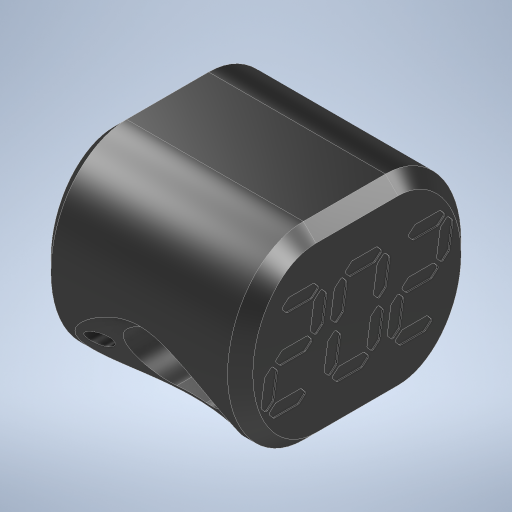
# Autodesk Inventor part: HeadCover
Saved by Autodesk Inventor 2024.2 (Build 282272000, 272)
## iProperties
Created: 2024-02-01
Part Number: HeadCover
Material: ABS Plastic
Document SubType Name: Modeling
Designer: Masato Kubotera
Density: 1.06 g/cm^3
Appearance: Glossy - Black
Mass: 122.703 g
Surface Area: 426.62 cm^2
Volume: 115.757 cm^3
Catalog Web Link: https://www.poly-maker.jp/polyterra-pla.html
Author: Masato Kubotera
Autodesk Inventor part; units mm, degrees
ref_plane "YZ Plane" through (0, 0, 0) normal (1, 0, 0) x (0, 1, 0)
ref_plane "XZ Plane" through (0, 0, 0) normal (0, 1, 0) x (-1, 0, 0)
ref_plane "XY Plane" through (0, 0, 0) normal (0, 0, 1) x (1, 0, 0)
derived "HeadSideFrame.ipt"
sketch "Sketch1" plane through (0, 30, 0) normal (0, 1, 0) x (-1, 0, 0)
  line L0 (-53.8277, 71.1723) -> (-50.2922, 74.7078) construction
  line L1 (-46.0495, 70.4652) -> (-54.5348, 78.9505) construction
  line L2 (-46.0495, 70.4652) -> (-58.0704, 75.4149) construction
  line L3 (-46.0142, 70.4298) -> (-54.5702, 78.9858)
  arc A0 (-47.5142, 68.9298) -> (-47.5142, 71.9298) centre (-47.5142, 70.4298) ccw
  line L4 (-60.5452, 81.4253) -> (-43.5747, 64.4548) construction
  line L5 (-62.6665, 83.5467) -> (-41.4533, 62.3335) construction
  line L6 (-54.5348, 78.9505) -> (-49.5851, 66.9296) construction
  line L7 (-58.0704, 75.4149) -> (-49.5851, 66.9296) construction
  ellipse E0 centre (-46.25, 64.5) end of major axis (-46.25, 102) minor radius 30 (-46.25, 102) -> (-46.25, 27) ccw
  line L8 (-58.0704, 78.9505) -> (-74.7581, 62.2627) construction
  line L9 (-62.7373, 50.2419) -> (-46.0495, 66.9296) construction
  line L10 (-54.5348, 78.9505) -> (-58.0704, 75.4149) construction
  line L11 (-54.5702, 78.9858) -> (-58.7421, 74.8139)
  line L12 (-33.1802, 70.6066) -> (-54.3934, 91.8198) construction
  arc A1 (-53.0702, 77.4858) -> (-56.0702, 77.4858) centre (-54.5702, 77.4858) ccw
  line L13 (-7.3, -1.5) -> (-7.3, 3.5)
  line L14 (-46.25, 27) -> (-13.75, 27)
  line L15 (-7.25, -1.5) -> (-7.25, 3.5) construction
  line L16 (-41.4533, 62.3335) -> (-33.1802, 70.6066) construction
  line L17 (-49.5851, 66.9296) -> (-46.0495, 70.4652) construction
  line L18 (-54.3934, 91.8198) -> (-62.6665, 83.5467) construction
  line L19 (-46.25, 102) -> (-46.25, 27) construction
  line L20 (-30, 102) -> (-30, 27) construction
  line L21 (-46.25, 102) -> (-13.75, 102)
  line L22 (10.1236, 102) -> (65.1439, 102) construction
  ellipse E1 centre (-13.75, 64.5) end of major axis (-13.75, 102) minor radius 30 (-13.75, 27) -> (-13.75, 102) ccw
  line L23 (-16.25, -1.5) -> (16.25, -1.5)
  arc A2 (-4.3, 3.5) -> (-7.3, 3.5) centre (-5.8, 3.5) ccw
  line L24 (0, -1.5) -> (0, 3.5) construction
  line L25 (-7.3, 3.5) -> (7.3, 3.5)
  arc A3 (7.3, 3.5) -> (4.3, 3.5) centre (5.8, 3.5) ccw
  line L26 (-13.25, 1) -> (13.25, 1) construction
  line L27 (7.25, -1.5) -> (7.25, 3.5) construction
  line L28 (7.3, 3.5) -> (7.3, -1.5)
  line L29 (0, 0) -> (-125, 0) construction
  line L30 (-65, 60) -> (-125, 0) construction
  line L31 (-74.7581, 62.2627) -> (-62.7373, 50.2419) construction
  line L32 (-58.9896, 53.9896) -> (-71.0104, 66.0104) construction
  line L33 (-57.5883, 37.2154) -> (-87.7846, 67.4117) construction
  line L34 (-65, 60) -> (-57.5883, 37.2154) construction
  line L35 (-65, 60) -> (-87.7846, 67.4117) construction
  line L36 (-46.0142, 70.4298) -> (-50.1861, 66.2579)
  line L37 (-58.7421, 74.8139) -> (-68.1169, 84.1887)
  line L38 (16.25, -1.5) -> (16.25, 64.5)
  line L39 (-16.25, -1.5) -> (-16.25, 27)
  line L40 (-30.419, 89.6005) -> (-26.8835, 93.136) construction
  line L41 (-26.8835, 93.136) -> (9.886, 56.3665) construction
  line L42 (9.886, 56.3665) -> (6.3505, 52.831) construction
  line L43 (6.3505, 52.831) -> (-30.419, 89.6005) construction
  line L44 (-30.419, 89.6005) -> (9.886, 56.3665) construction
  line L45 (-26.8835, 93.136) -> (6.3505, 52.831) construction
  line L46 (-30.4898, 89.6005) -> (-26.8835, 93.2067)
  line L47 (-30.4898, 89.6005) -> (9.9567, 56.3665) construction
  line L48 (-26.8835, 93.2067) -> (9.9567, 56.3665)
  line L49 (9.9567, 56.3665) -> (6.3505, 52.7602)
  line L50 (6.3505, 52.7602) -> (-30.4898, 89.6005)
  line L51 (-26.8835, 93.2067) -> (6.3505, 52.7602) construction
  arc A4 (-24.7622, 91.0854) -> (-26.8835, 93.2067) centre (-25.8229, 92.1461) ccw
  line L52 (-35.0152, 97.7322) -> (14.4822, 48.2348) construction
  line L53 (-8.4634, 74.7866) -> (-12.0696, 71.1804) construction
  arc A5 (-30.4898, 89.6005) -> (-28.3684, 87.4792) centre (-29.4291, 88.5398) ccw
  arc A6 (4.2292, 54.8816) -> (6.3505, 52.7602) centre (5.2898, 53.8209) ccw
  arc A7 (9.9567, 56.3665) -> (7.8354, 58.4878) centre (8.8961, 57.4271) ccw
  line L54 (-46.25, 56.7553) -> (-46.25, 27)
  line L55 (-33.2475, 99.5) -> (-36.783, 95.9645) construction
  line L56 (-40.35, 36) -> (-46.25, 36) construction
  line L57 (-46.25, 48) -> (-40.35, 48) construction
  line L58 (-40.35, 48) -> (-40.35, 36) construction
  line L59 (-40.35, 36) -> (-46.25, 48) construction
  line L60 (-46.25, 36) -> (-40.35, 48) construction
  line L61 (-46.25, 48.05) -> (-40.35, 48.05)
  line L62 (-40.35, 48.05) -> (-40.35, 35.95)
  line L63 (-40.35, 35.95) -> (-46.25, 35.95)
  line L64 (-40.35, 42) -> (-46.25, 42) construction
  arc A8 (-40.35, 45.05) -> (-40.35, 48.05) centre (-40.35, 46.55) ccw
  line L65 (-42.85, 54) -> (-42.85, 30) construction
  line L66 (-46.25, 57) -> (-40.35, 57) construction
  arc A9 (-40.35, 35.95) -> (-40.35, 38.95) centre (-40.35, 37.45) ccw
  line L67 (-65.0707, 81.1425) -> (-60.8988, 85.3144) construction
  line L68 (-43.2211, 60.5657) -> (-39.6856, 64.1012) construction
  line L69 (-46.25, 64.5) -> (-76.25, 64.5) construction
  line L70 (-13.75, 64.5) -> (16.25, 64.5) construction
  line L71 (-11.75, 8) -> (11.75, 8)
  line L72 (-46.25, 99.5) -> (-13.75, 99.5)
  line L73 (-50.1861, 66.2579) -> (-46.25, 70.194)
  circle A10 centre (-42.85, 30) radius 2.4 construction
  circle A11 centre (-60.5452, 81.4253) radius 2.4 construction
  line L74 (-50.1861, 66.2579) -> (-50.1861, 66.2579)
  line L75 (4.9456, 48.5083) -> (-23.7522, 77.2061)
  line L76 (-26.5807, 77.2061) -> (-35.7642, 68.0226)
  line L77 (-36.35, 66.6084) -> (-36.35, 31.5)
  line L78 (-28.3484, 81.8023) -> (-43.1484, 96.6023)
  line L79 (-28.3484, 78.9739) -> (-37.9607, 69.3616)
  line L80 (-40.7891, 69.3616) -> (-57.284, 85.8565)
  line L81 (-18.7392, 29.5) -> (-34.35, 29.5)
  line L82 (9.4147, 83.2799) -> (16.25, 64.5)
  line L83 (-13.75, 102) -> (-13.75, 27) construction
  line L84 (-13.75, 99.5) -> (9.4147, 83.2799)
  line L85 (16.25, 64.5) -> (9.4147, 45.7201)
  line L86 (9.4147, 45.7201) -> (-12.8972, 30.0972)
  line L87 (-46.25, 27) -> (-16.25, 27)
  line L88 (-13.75, 28.4589) -> (-13.75, 10)
  line L89 (13.75, 10) -> (13.75, 44.9137)
  line L90 (-46.25, 99.5) -> (-68.1169, 84.1887)
  line L91 (9.4147, 45.7201) -> (10.6028, 46.552)
  line L92 (4.6786, 45.4558) -> (-17.5921, 29.8617)
  line L93 (-57.0169, 88.909) -> (-45.7097, 96.8264)
  arc A12 (-43.1484, 96.6023) -> (-45.7097, 96.8264) centre (-44.5626, 95.1881) ccw
  arc A13 (-57.0169, 88.909) -> (-57.284, 85.8565) centre (-55.8698, 87.2707) ccw
  arc A14 (-40.7891, 69.3616) -> (-37.9607, 69.3616) centre (-39.3749, 70.7758) ccw
  arc A15 (-28.3484, 78.9739) -> (-28.3484, 81.8023) centre (-29.7626, 80.3881) ccw
  arc A16 (-23.7522, 77.2061) -> (-26.5807, 77.2061) centre (-25.1665, 75.7919) ccw
  arc A17 (4.6786, 45.4558) -> (4.9456, 48.5083) centre (3.5314, 47.0941) ccw
  arc A18 (-18.7392, 29.5) -> (-17.5921, 29.8617) centre (-18.7392, 31.5) ccw
  arc A19 (-36.35, 31.5) -> (-34.35, 29.5) centre (-34.35, 31.5) ccw
  arc A20 (-35.7642, 68.0226) -> (-36.35, 66.6084) centre (-34.35, 66.6084) ccw
  arc A21 (13.75, 44.9137) -> (10.6028, 46.552) centre (11.75, 44.9137) ccw
  arc A22 (-12.8972, 30.0972) -> (-13.75, 28.4589) centre (-11.75, 28.4589) ccw
  arc A23 (-13.75, 10) -> (-11.75, 8) centre (-11.75, 10) ccw
  arc A24 (11.75, 8) -> (13.75, 10) centre (11.75, 10) ccw
  arc A25 (-46.25, 56.7553) -> (-50.1861, 66.2579) centre (-59.6887, 56.7553) ccw
  line L94 (12.7145, 46.467) -> (16.25, 50.0025) construction
  point P0 (-52.0599, 72.9401)
  point P1 (-72.6865, 52.3135)
  point P2 (-10.2665, 72.9835)
  point P3 (-46.25, 62.3218)
  point P4 (-32.8939, 95.6109)
  point P5 (12.3609, 50.3561)
  point P6 (-43.3, 42)
  point P7 (-73.75, 64.5)
  point P8 (-13.75, 8)
  point P9 (13.75, 8)
  point P10 (6.631, 46.8229)
  point P11 (-25.1665, 78.6203)
  point P12 (-36.35, 67.4368)
  point P13 (-36.35, 29.5)
  point P14 (-26.9342, 80.3881)
  point P15 (-44.335, 97.7889)
  point P16 (-71.25, 64.5)
  point P17 (-39.3749, 67.9474)
  point P18 (-58.9694, 87.5419)
  point P19 (-13.75, 29.5)
  point P20 (13.75, 57.6313)
  point P21 (13.75, 48.7557)
  point P22 (-18.1086, 29.5)
sketch "Sketch2" plane through (0, 0, 0) normal (0, 1, 0) x (-1, 0, 0)
  ellipse E0 centre (-46.25, 64.5) end of major axis (-46.25, 102) minor radius 30 (-46.25, 102) -> (-46.25, 27) ccw projected
  ellipse E1 centre (-13.75, 64.5) end of major axis (-13.75, 102) minor radius 30 (-13.75, 27) -> (-13.75, 102) ccw projected
  line L0 (-46.25, 27) -> (-13.75, 27) projected
  line L1 (-65, 60) -> (-53.0561, 23.2827)
  line L2 (-53.0561, 23.2827) -> (-101.7173, 71.9439)
  line L3 (-101.7173, 71.9439) -> (-65, 60)
  line L4 (-65, 60) -> (-87.7846, 67.4117) construction
  line L5 (-65, 60) -> (-57.5883, 37.2154) construction
  line L6 (-74.7581, 62.2627) -> (-62.7373, 50.2419) construction
  line L7 (-65, 60) -> (-77.3867, 47.6133)
  line L8 (-46.25, 102) -> (-13.75, 102) projected
  line L9 (-46.6859, 99.5) -> (-13.3141, 99.5)
  line L10 (-13.3141, 99.5) -> (13.2213, 80.9197)
  line L11 (-46.25, 99.5) -> (-13.75, 99.5) projected
  line L12 (-13.75, 99.5) -> (9.4147, 83.2799) projected
  line L13 (-30, 102) -> (-30, 27) construction
  line L14 (-46.6859, 99.5) -> (-68.5043, 84.2226)
  arc A0 (-46.25, 56.7553) -> (-50.1861, 66.2579) centre (-59.6887, 56.7553) ccw projected
  line L15 (-46.25, 56.7553) -> (-46.25, 27) projected
  line L16 (-68.5043, 84.2226) -> (-50.3629, 66.0811)
  line L17 (-46.5, 27.0013) -> (-46.5, 56.7553)
  line L18 (-58.7421, 74.8139) -> (-68.1169, 84.1887) projected
  arc A1 (-46.5, 56.7553) -> (-50.3629, 66.0811) centre (-59.6887, 56.7553) ccw
  line L19 (-46.25, 64.5) -> (-76.25, 64.5) construction
  point P0 (0, 0)
  point P1 (16.25, 64.5)
  point P2 (-64.9909, 35.2174)
  point P3 (-46.5, 27)
  point P4 (-76.2424, 63.6571)
  point P5 (-54.7673, 28.5431)
  dimension "d70" = 0.25
  dimension "d78" = 0.25
  dimension "d79" = 0.25
  dimension "d99" = 29.75
  constraints: 19 end point, 3 collinear, 3 parallel, 3 point on line, 2 point on circle, 1 centre point, 1 coincident, 1 concentric, 1 horizontal, 1 midpoint, 1 tangent, 1 vertical, 7 other
  measures "d70" distance between parallel lines of L12 L10
  measures "d78" distance from line of point (-46.5, 27) L15
  measures "d79" distance between parallel lines of L16 L18
  measures "d99" distance from line of point (-76.25, 64.5) L17
extrude "Extrusion1" add sketch "Sketch2" along normal blind 40 contours L17 A1 L16 L14 L9 L10 E1 L0 E0 | E0 L1 L3 L8 E1 L10 L9 L14 L16 A1 L17 | E0 L7 L1 | L7 E0 L3
revolve "Revolution1" cut sketch "Sketch2" angle 360 about axis through (65, 0, 60) along (0.7071068, 0, -0.7071068) contours L7 E0 L3 | L7 L2 L3 E0
ref_plane "Work Plane1" through (64.9909, 0, 35.2174) normal (0.7071068, 0, -0.7071068) x (0, 1, 0)
ref_plane "Work Plane2" through (76.25, 0, 64.5) normal (1, 0, 0) x (0, 1, 0)
sketch "Sketch3" plane through (64.9909, 0, 35.2174) normal (0.7071068, 0, -0.7071068) x (0, 1, 0)
  arc A0 (10, 17.5304) -> (-10, 17.5304) centre (0, 17.5304) ccw
  line L0 (-10, 17.5304) -> (-10, -0.4696)
  arc A1 (-10, -0.4696) -> (10, -0.4696) centre (0, -0.4696) ccw
  line L1 (0, -16.8783) -> (0, 51.9391) construction
  line L2 (-10, 8.5304) -> (8.9009, 8.5304) construction
  line L3 (10, 17.5304) -> (10, -0.4696)
  point P0 (0, -70.8579)
  dimension "d80" = 20
  dimension "d81" = 18
  constraints: 6 end point, 4 point on circle, 2 centre point, 2 symmetric about line, 1 coincident, 1 horizontal, 1 midpoint, 1 point on line, 1 tangent, 1 vertical, 1 other
  measures "d80" diameter of A0
  measures "d81" distance of A1.centre point (0, 17.53)
extrude "Extrusion2" cut sketch "Sketch2" along normal blind 33 contours L17 A1 L16 L14 L9 L10 E1 L0 E0
extrude "Extrusion3" cut sketch "Sketch3" against normal up to surface (32.1675 mm away)
sketch "Sketch4" plane through (76.25, 0, 64.5) normal (1, 0, 0) x (0, 1, 0)
  arc A0 (5.85, -34.65) -> (5.85, -10.35) centre (5.85, -22.5) ccw
  line L0 (5.85, -10.35) -> (-5.85, -10.35)
  line L1 (5.85, -34.65) -> (-5.85, -34.65)
  line L2 (0, -10.35) -> (0, -34.65) construction
  arc A1 (-5.85, -10.35) -> (-5.85, -34.65) centre (-5.85, -22.5) ccw
  line L3 (-5.85, -22.5) -> (5.85, -22.5) construction
  point P0 (0, -64.5)
  point P1 (30, -22.5)
  point P2 (30, -22.5)
  point P3 (30, -22.5)
  point P4 (25, -22.5)
  point P5 (-25, -22.5)
  dimension "d84" = 24.3
  dimension "d85" = 11.7
  dimension "d91" = 50
  constraints: 8 end point, 4 point on circle, 4 point on line, 3 horizontal, 2 centre point, 2 midpoint, 2 symmetric about line, 2 tangent, 1 vertical, 1 other
  measures "d84" diameter of A0
  measures "d85" distance of L3.end L3.start
  measures "d91" distance of point (25, -22.5) point (-25, -22.5)
extrude "Extrusion4" cut sketch "Sketch4" against normal up to surface (29.75 mm away)
chamfer "C5" distance 5 angle 45 4 edges at (76.25, 40, 64.5) (30, 40, 27) (-16.25, 40, 64.5) (30, 40, 102)
hole "Phi3.5" at (76.25, 25, 42) at (76.25, -25, 42) direction (-1, 0, 0) diameter 3.5 depth 29.75 counterbore diameter 7.5 counterbore depth 24.75
mirror "Mirror1" about plane through (0, 0, 0) normal (0, 1, 0)
fillet "R2" radius 2 1 edges at (68.5043, 0, 84.2226)
sketch "Sketch14" plane through (0, 40, 0) normal (0, 1, 0) x (1, 0, 0)
  line L0 (30.3514, -62) -> (29.6486, -67) construction
  line L1 (24.9893, -67) -> (34.308, -67)
  arc A0 (24.42, -66.7383) -> (24.9893, -67) centre (24.9893, -66.25) ccw
  arc A1 (24.3659, -61.2041) -> (24.6189, -60.749) centre (23.8776, -60.6349) ccw
  line L2 (25.2037, -62.1807) -> (23.0693, -64.0117)
  line L3 (22.9883, -65.0693) -> (24.42, -66.7383)
  arc A2 (23.0693, -64.0117) -> (22.9883, -65.0693) centre (23.5576, -64.5809) ccw
  line L4 (24.3659, -61.2041) -> (22.2315, -63.0351)
  arc A3 (21.1739, -62.9541) -> (22.2315, -63.0351) centre (21.7432, -62.4658) ccw
  line L5 (25.692, -62) -> (35.0107, -62)
  arc A4 (41.3422, -61.2041) -> (41.5952, -60.749) centre (40.8539, -60.6349) ccw
  line L6 (38.8261, -66.0459) -> (40.2578, -67.7149)
  line L7 (41.3422, -61.2041) -> (39.2078, -63.0351)
  arc A5 (38.1502, -62.9541) -> (39.2078, -63.0351) centre (38.7195, -62.4658) ccw
  arc A6 (43.0133, -51.5388) -> (42.8413, -50.9364) centre (42.272, -51.4247) ccw
  line L8 (43.0133, -51.5388) -> (41.5952, -60.749)
  arc A7 (36.9307, -64.9883) -> (37.0117, -63.9307) centre (36.4424, -64.4191) ccw
  line L9 (38.1502, -62.9541) -> (36.7185, -61.2851)
  arc A8 (36.5465, -60.6826) -> (36.7185, -61.2851) centre (37.2877, -60.7968) ccw
  arc A9 (38.2175, -51.0173) -> (37.9646, -51.4725) centre (38.7058, -51.5866) ccw
  line L10 (37.9646, -51.4725) -> (36.5465, -60.6826)
  arc A10 (38.8261, -66.0459) -> (37.7685, -65.9649) centre (38.2568, -66.5342) ccw
  line L11 (26.037, -51.5388) -> (24.6189, -60.749)
  line L12 (23.945, -48.6981) -> (21.6622, -63.5234) construction
  line L13 (20.9883, -51.4725) -> (19.5702, -60.6826)
  arc A11 (25.692, -62) -> (25.2037, -62.1807) centre (25.692, -62.75) ccw
  arc A12 (19.5702, -60.6826) -> (19.7422, -61.2851) centre (20.3114, -60.7968) ccw
  line L14 (21.1739, -62.9541) -> (19.7422, -61.2851)
  arc A13 (16.9867, -77.4612) -> (17.1587, -78.0636) centre (17.728, -77.5753) ccw
  line L15 (21.7825, -77.9827) -> (19.648, -79.8136)
  arc A14 (18.5905, -79.7327) -> (19.648, -79.8136) centre (19.1597, -79.2443) ccw
  line L16 (18.5905, -79.7327) -> (17.1587, -78.0636)
  line L17 (18.4048, -68.251) -> (16.9867, -77.4612)
  arc A15 (18.6578, -67.7959) -> (18.4048, -68.251) centre (19.1461, -68.3651) ccw
  line L18 (23.4535, -68.3174) -> (22.0354, -77.5275)
  line L19 (20.7922, -65.9649) -> (18.6578, -67.7959)
  arc A16 (21.8498, -66.0459) -> (20.7922, -65.9649) centre (21.2805, -66.5342) ccw
  arc A17 (23.4535, -68.3174) -> (23.2815, -67.7149) centre (22.7123, -68.2032) ccw
  line L20 (21.8498, -66.0459) -> (23.2815, -67.7149)
  arc A18 (21.7825, -77.9827) -> (22.0354, -77.5275) centre (21.2942, -77.4134) ccw
  arc A19 (31.7245, -83.7785) -> (32.2128, -83.5978) centre (31.7245, -83.0285) ccw
  line L21 (23.1085, -78.7785) -> (32.4272, -78.7785)
  arc A20 (23.1085, -78.7785) -> (22.6202, -78.9593) centre (23.1085, -79.5285) ccw
  line L22 (22.4058, -83.7785) -> (31.7245, -83.7785)
  arc A21 (21.8366, -83.5169) -> (22.4058, -83.7785) centre (22.4058, -83.0285) ccw
  line L23 (20.4048, -81.8478) -> (21.8366, -83.5169)
  arc A22 (20.4858, -80.7902) -> (20.4048, -81.8478) centre (20.9741, -81.3595) ccw
  line L24 (22.6202, -78.9593) -> (20.4858, -80.7902)
  line L25 (41.4095, -49.2673) -> (42.8413, -50.9364)
  arc A23 (41.4095, -49.2673) -> (40.352, -49.1864) centre (40.8403, -49.7557) ccw
  line L26 (38.1634, -45.4831) -> (39.5952, -47.1522)
  line L27 (40.352, -49.1864) -> (38.2175, -51.0173)
  line L28 (37.3798, -50.0407) -> (39.5142, -48.2098)
  arc A24 (36.8915, -50.2215) -> (37.3798, -50.0407) centre (36.8915, -49.4715) ccw
  arc A25 (39.5142, -48.2098) -> (39.5952, -47.1522) centre (39.0259, -47.6405) ccw
  arc A26 (21.2413, -51.0173) -> (20.9883, -51.4725) centre (21.7296, -51.5866) ccw
  arc A27 (26.037, -51.5388) -> (25.865, -50.9364) centre (25.2958, -51.4247) ccw
  line L29 (23.3757, -49.1864) -> (21.2413, -51.0173)
  line L30 (24.4333, -49.2673) -> (25.865, -50.9364)
  arc A28 (24.4333, -49.2673) -> (23.3757, -49.1864) centre (23.864, -49.7557) ccw
  arc A29 (38.1634, -45.4831) -> (37.5942, -45.2215) centre (37.5942, -45.9715) ccw
  line L31 (28.2755, -45.2215) -> (37.5942, -45.2215)
  line L32 (40.0835, -47.7215) -> (25.0835, -47.7215) construction
  line L33 (27.5728, -50.2215) -> (36.8915, -50.2215)
  arc A30 (28.2755, -45.2215) -> (27.7872, -45.4022) centre (28.2755, -45.9715) ccw
  arc A31 (27.0035, -49.9598) -> (27.5728, -50.2215) centre (27.5728, -49.4715) ccw
  line L34 (27.7872, -45.4022) -> (25.6527, -47.2331)
  line L35 (25.5718, -48.2907) -> (27.0035, -49.9598)
  arc A32 (25.6527, -47.2331) -> (25.5718, -48.2907) centre (26.141, -47.8024) ccw
  arc A33 (35.58, -62.2617) -> (35.0107, -62) centre (35.0107, -62.75) ccw
  line L36 (35.58, -62.2617) -> (37.0117, -63.9307)
  arc A34 (34.308, -67) -> (34.7963, -66.8193) centre (34.308, -66.25) ccw
  arc A35 (35.6341, -67.7959) -> (35.3811, -68.251) centre (36.1224, -68.3651) ccw
  line L37 (34.7963, -66.8193) -> (36.9307, -64.9883)
  line L38 (37.7685, -65.9649) -> (35.6341, -67.7959)
  arc A36 (40.4298, -68.3174) -> (40.2578, -67.7149) centre (39.6886, -68.2032) ccw
  arc A37 (32.9965, -79.0402) -> (32.4272, -78.7785) centre (32.4272, -79.5285) ccw
  line L39 (32.2128, -83.5978) -> (34.3473, -81.7669)
  line L40 (32.9965, -79.0402) -> (34.4282, -80.7093)
  arc A38 (34.3473, -81.7669) -> (34.4282, -80.7093) centre (33.859, -81.1976) ccw
  line L41 (35.3811, -68.251) -> (33.963, -77.4612)
  line L42 (40.4298, -68.3174) -> (39.0117, -77.5275)
  arc A39 (33.963, -77.4612) -> (34.135, -78.0636) centre (34.7042, -77.5753) ccw
  line L43 (38.7587, -77.9827) -> (36.6243, -79.8136)
  line L44 (35.5667, -79.7327) -> (34.135, -78.0636)
  arc A40 (35.5667, -79.7327) -> (36.6243, -79.8136) centre (36.136, -79.2443) ccw
  arc A41 (38.7587, -77.9827) -> (39.0117, -77.5275) centre (38.2704, -77.4134) ccw
  line L45 (46.25, -97) -> (13.75, -97) projected
  line L46 (30, -97) -> (30, -32) construction
  line L47 (13.75, -32) -> (46.25, -32) projected
  line L48 (5.3514, -62) -> (4.6486, -67) construction
  line L49 (0.692, -62) -> (10.0107, -62)
  line L50 (-0.0107, -67) -> (9.308, -67)
  arc A42 (2.0035, -49.9598) -> (2.5728, -50.2215) centre (2.5728, -49.4715) ccw
  line L51 (12.9646, -51.4725) -> (11.5465, -60.6826)
  arc A43 (13.2175, -51.0173) -> (12.9646, -51.4725) centre (13.7058, -51.5866) ccw
  line L52 (18.0133, -51.5388) -> (16.5952, -60.749)
  line L53 (2.5728, -50.2215) -> (11.8915, -50.2215)
  line L54 (15.352, -49.1864) -> (13.2175, -51.0173)
  arc A44 (16.3422, -61.2041) -> (16.5952, -60.749) centre (15.8539, -60.6349) ccw
  line L55 (16.3422, -61.2041) -> (14.2078, -63.0351)
  arc A45 (13.1502, -62.9541) -> (14.2078, -63.0351) centre (13.7195, -62.4658) ccw
  arc A46 (13.8261, -66.0459) -> (12.7685, -65.9649) centre (13.2568, -66.5342) ccw
  line L56 (13.8261, -66.0459) -> (15.2578, -67.7149)
  line L57 (-2.0117, -65.0693) -> (-0.58, -66.7383)
  line L58 (-3.1502, -66.0459) -> (-1.7185, -67.7149)
  arc A47 (-1.5465, -68.3174) -> (-1.7185, -67.7149) centre (-2.2877, -68.2032) ccw
  arc A48 (-0.58, -66.7383) -> (-0.0107, -67) centre (-0.0107, -66.25) ccw
  arc A49 (-3.1502, -66.0459) -> (-4.2078, -65.9649) centre (-3.7195, -66.5342) ccw
  line L59 (-4.2078, -65.9649) -> (-6.3422, -67.7959)
  arc A50 (-6.3422, -67.7959) -> (-6.5952, -68.251) centre (-5.8539, -68.3651) ccw
  line L60 (-6.5952, -68.251) -> (-8.0133, -77.4612)
  line L61 (-1.5465, -68.3174) -> (-2.9646, -77.5275)
  line L62 (0.5718, -48.2907) -> (2.0035, -49.9598)
  arc A51 (1.037, -51.5388) -> (0.865, -50.9364) centre (0.2958, -51.4247) ccw
  line L63 (-0.5667, -49.2673) -> (0.865, -50.9364)
  line L64 (-1.6243, -49.1864) -> (-3.7587, -51.0173)
  line L65 (1.037, -51.5388) -> (-0.3811, -60.749)
  arc A52 (-3.7587, -51.0173) -> (-4.0117, -51.4725) centre (-3.2704, -51.5866) ccw
  arc A53 (0.692, -62) -> (0.2037, -62.1807) centre (0.692, -62.75) ccw
  arc A54 (-0.6341, -61.2041) -> (-0.3811, -60.749) centre (-1.1224, -60.6349) ccw
  line L66 (-1.055, -48.6981) -> (-3.3378, -63.5234) construction
  line L67 (-4.0117, -51.4725) -> (-5.4298, -60.6826)
  arc A55 (-1.9307, -64.0117) -> (-2.0117, -65.0693) centre (-1.4424, -64.5809) ccw
  line L68 (-0.6341, -61.2041) -> (-2.7685, -63.0351)
  line L69 (0.2037, -62.1807) -> (-1.9307, -64.0117)
  arc A56 (-3.8261, -62.9541) -> (-2.7685, -63.0351) centre (-3.2568, -62.4658) ccw
  arc A57 (10.58, -62.2617) -> (10.0107, -62) centre (10.0107, -62.75) ccw
  arc A58 (11.5465, -60.6826) -> (11.7185, -61.2851) centre (12.2877, -60.7968) ccw
  line L70 (13.1502, -62.9541) -> (11.7185, -61.2851)
  line L71 (10.58, -62.2617) -> (12.0117, -63.9307)
  line L72 (9.7963, -66.8193) -> (11.9307, -64.9883)
  arc A59 (11.9307, -64.9883) -> (12.0117, -63.9307) centre (11.4424, -64.4191) ccw
  arc A60 (-5.4298, -60.6826) -> (-5.2578, -61.2851) centre (-4.6886, -60.7968) ccw
  line L73 (-3.8261, -62.9541) -> (-5.2578, -61.2851)
  arc A61 (8.963, -77.4612) -> (9.135, -78.0636) centre (9.7042, -77.5753) ccw
  arc A62 (9.308, -67) -> (9.7963, -66.8193) centre (9.308, -66.25) ccw
  line L74 (10.3811, -68.251) -> (8.963, -77.4612)
  arc A63 (10.6341, -67.7959) -> (10.3811, -68.251) centre (11.1224, -68.3651) ccw
  line L75 (10.5667, -79.7327) -> (9.135, -78.0636)
  line L76 (13.7587, -77.9827) -> (11.6243, -79.8136)
  line L77 (15.4298, -68.3174) -> (14.0117, -77.5275)
  line L78 (12.7685, -65.9649) -> (10.6341, -67.7959)
  arc A64 (15.4298, -68.3174) -> (15.2578, -67.7149) centre (14.6886, -68.2032) ccw
  arc A65 (18.0133, -51.5388) -> (17.8413, -50.9364) centre (17.272, -51.4247) ccw
  arc A66 (13.1634, -45.4831) -> (12.5942, -45.2215) centre (12.5942, -45.9715) ccw
  line L79 (13.1634, -45.4831) -> (14.5952, -47.1522)
  arc A67 (14.5142, -48.2098) -> (14.5952, -47.1522) centre (14.0259, -47.6405) ccw
  line L80 (12.3798, -50.0407) -> (14.5142, -48.2098)
  arc A68 (16.4095, -49.2673) -> (15.352, -49.1864) centre (15.8403, -49.7557) ccw
  line L81 (16.4095, -49.2673) -> (17.8413, -50.9364)
  arc A69 (11.8915, -50.2215) -> (12.3798, -50.0407) centre (11.8915, -49.4715) ccw
  arc A70 (-1.8915, -78.7785) -> (-2.3798, -78.9593) centre (-1.8915, -79.5285) ccw
  line L82 (-1.8915, -78.7785) -> (7.4272, -78.7785)
  arc A71 (6.7245, -83.7785) -> (7.2128, -83.5978) centre (6.7245, -83.0285) ccw
  arc A72 (7.9965, -79.0402) -> (7.4272, -78.7785) centre (7.4272, -79.5285) ccw
  line L83 (7.2128, -83.5978) -> (9.3473, -81.7669)
  line L84 (7.9965, -79.0402) -> (9.4282, -80.7093)
  arc A73 (9.3473, -81.7669) -> (9.4282, -80.7093) centre (8.859, -81.1976) ccw
  arc A74 (10.5667, -79.7327) -> (11.6243, -79.8136) centre (11.136, -79.2443) ccw
  line L85 (-2.5942, -83.7785) -> (6.7245, -83.7785)
  arc A75 (-4.5142, -80.7902) -> (-4.5952, -81.8478) centre (-4.0259, -81.3595) ccw
  line L86 (-4.5952, -81.8478) -> (-3.1634, -83.5169)
  arc A76 (13.7587, -77.9827) -> (14.0117, -77.5275) centre (13.2704, -77.4134) ccw
  arc A77 (-3.1634, -83.5169) -> (-2.5942, -83.7785) centre (-2.5942, -83.0285) ccw
  arc A78 (-3.2175, -77.9827) -> (-2.9646, -77.5275) centre (-3.7058, -77.4134) ccw
  line L87 (-2.3798, -78.9593) -> (-4.5142, -80.7902)
  line L88 (-3.2175, -77.9827) -> (-5.352, -79.8136)
  arc A79 (-6.4095, -79.7327) -> (-5.352, -79.8136) centre (-5.8403, -79.2443) ccw
  line L89 (-6.4095, -79.7327) -> (-7.8413, -78.0636)
  arc A80 (-8.0133, -77.4612) -> (-7.8413, -78.0636) centre (-7.272, -77.5753) ccw
  line L90 (15.0835, -47.7215) -> (0.0835, -47.7215) construction
  line L91 (3.2755, -45.2215) -> (12.5942, -45.2215)
  arc A81 (3.2755, -45.2215) -> (2.7872, -45.4022) centre (3.2755, -45.9715) ccw
  line L92 (2.7872, -45.4022) -> (0.6527, -47.2331)
  arc A82 (0.6527, -47.2331) -> (0.5718, -48.2907) centre (1.141, -47.8024) ccw
  arc A83 (-0.5667, -49.2673) -> (-1.6243, -49.1864) centre (-1.136, -49.7557) ccw
  line L93 (55.3514, -62) -> (54.6486, -67) construction
  line L94 (50.692, -62) -> (60.0107, -62)
  line L95 (49.9893, -67) -> (59.308, -67)
  arc A84 (52.0035, -49.9598) -> (52.5728, -50.2215) centre (52.5728, -49.4715) ccw
  line L96 (62.9646, -51.4725) -> (61.5465, -60.6826)
  arc A85 (63.2175, -51.0173) -> (62.9646, -51.4725) centre (63.7058, -51.5866) ccw
  line L97 (68.0133, -51.5388) -> (66.5952, -60.749)
  line L98 (52.5728, -50.2215) -> (61.8915, -50.2215)
  line L99 (65.352, -49.1864) -> (63.2175, -51.0173)
  arc A86 (66.3422, -61.2041) -> (66.5952, -60.749) centre (65.8539, -60.6349) ccw
  line L100 (66.3422, -61.2041) -> (64.2078, -63.0351)
  arc A87 (63.1502, -62.9541) -> (64.2078, -63.0351) centre (63.7195, -62.4658) ccw
  arc A88 (63.8261, -66.0459) -> (62.7685, -65.9649) centre (63.2568, -66.5342) ccw
  line L101 (63.8261, -66.0459) -> (65.2578, -67.7149)
  line L102 (47.9883, -65.0693) -> (49.42, -66.7383)
  line L103 (46.8498, -66.0459) -> (48.2815, -67.7149)
  arc A89 (48.4535, -68.3174) -> (48.2815, -67.7149) centre (47.7123, -68.2032) ccw
  arc A90 (49.42, -66.7383) -> (49.9893, -67) centre (49.9893, -66.25) ccw
  arc A91 (46.8498, -66.0459) -> (45.7922, -65.9649) centre (46.2805, -66.5342) ccw
  line L104 (45.7922, -65.9649) -> (43.6578, -67.7959)
  arc A92 (43.6578, -67.7959) -> (43.4048, -68.251) centre (44.1461, -68.3651) ccw
  line L105 (43.4048, -68.251) -> (41.9867, -77.4612)
  line L106 (48.4535, -68.3174) -> (47.0354, -77.5275)
  line L107 (50.5718, -48.2907) -> (52.0035, -49.9598)
  arc A93 (51.037, -51.5388) -> (50.865, -50.9364) centre (50.2958, -51.4247) ccw
  line L108 (49.4333, -49.2673) -> (50.865, -50.9364)
  line L109 (48.3757, -49.1864) -> (46.2413, -51.0173)
  line L110 (51.037, -51.5388) -> (49.6189, -60.749)
  arc A94 (46.2413, -51.0173) -> (45.9883, -51.4725) centre (46.7296, -51.5866) ccw
  arc A95 (50.692, -62) -> (50.2037, -62.1807) centre (50.692, -62.75) ccw
  arc A96 (49.3659, -61.2041) -> (49.6189, -60.749) centre (48.8776, -60.6349) ccw
  line L111 (48.945, -48.6981) -> (46.6622, -63.5234) construction
  line L112 (45.9883, -51.4725) -> (44.5702, -60.6826)
  arc A97 (48.0693, -64.0117) -> (47.9883, -65.0693) centre (48.5576, -64.5809) ccw
  line L113 (49.3659, -61.2041) -> (47.2315, -63.0351)
  line L114 (50.2037, -62.1807) -> (48.0693, -64.0117)
  arc A98 (46.1739, -62.9541) -> (47.2315, -63.0351) centre (46.7432, -62.4658) ccw
  arc A99 (60.58, -62.2617) -> (60.0107, -62) centre (60.0107, -62.75) ccw
  arc A100 (61.5465, -60.6826) -> (61.7185, -61.2851) centre (62.2877, -60.7968) ccw
  line L115 (63.1502, -62.9541) -> (61.7185, -61.2851)
  line L116 (60.58, -62.2617) -> (62.0117, -63.9307)
  line L117 (59.7963, -66.8193) -> (61.9307, -64.9883)
  arc A101 (61.9307, -64.9883) -> (62.0117, -63.9307) centre (61.4424, -64.4191) ccw
  arc A102 (44.5702, -60.6826) -> (44.7422, -61.2851) centre (45.3114, -60.7968) ccw
  line L118 (46.1739, -62.9541) -> (44.7422, -61.2851)
  arc A103 (58.963, -77.4612) -> (59.135, -78.0636) centre (59.7042, -77.5753) ccw
  arc A104 (59.308, -67) -> (59.7963, -66.8193) centre (59.308, -66.25) ccw
  line L119 (60.3811, -68.251) -> (58.963, -77.4612)
  arc A105 (60.6341, -67.7959) -> (60.3811, -68.251) centre (61.1224, -68.3651) ccw
  line L120 (60.5667, -79.7327) -> (59.135, -78.0636)
  line L121 (63.7587, -77.9827) -> (61.6243, -79.8136)
  line L122 (65.4298, -68.3174) -> (64.0117, -77.5275)
  line L123 (62.7685, -65.9649) -> (60.6341, -67.7959)
  arc A106 (65.4298, -68.3174) -> (65.2578, -67.7149) centre (64.6886, -68.2032) ccw
  arc A107 (68.0133, -51.5388) -> (67.8413, -50.9364) centre (67.272, -51.4247) ccw
  arc A108 (63.1634, -45.4831) -> (62.5942, -45.2215) centre (62.5942, -45.9715) ccw
  line L124 (63.1634, -45.4831) -> (64.5952, -47.1522)
  arc A109 (64.5142, -48.2098) -> (64.5952, -47.1522) centre (64.0259, -47.6405) ccw
  line L125 (62.3798, -50.0407) -> (64.5142, -48.2098)
  arc A110 (66.4095, -49.2673) -> (65.352, -49.1864) centre (65.8403, -49.7557) ccw
  line L126 (66.4095, -49.2673) -> (67.8413, -50.9364)
  arc A111 (61.8915, -50.2215) -> (62.3798, -50.0407) centre (61.8915, -49.4715) ccw
  arc A112 (48.1085, -78.7785) -> (47.6202, -78.9593) centre (48.1085, -79.5285) ccw
  line L127 (48.1085, -78.7785) -> (57.4272, -78.7785)
  arc A113 (56.7245, -83.7785) -> (57.2128, -83.5978) centre (56.7245, -83.0285) ccw
  arc A114 (57.9965, -79.0402) -> (57.4272, -78.7785) centre (57.4272, -79.5285) ccw
  line L128 (57.2128, -83.5978) -> (59.3473, -81.7669)
  line L129 (57.9965, -79.0402) -> (59.4282, -80.7093)
  arc A115 (59.3473, -81.7669) -> (59.4282, -80.7093) centre (58.859, -81.1976) ccw
  arc A116 (60.5667, -79.7327) -> (61.6243, -79.8136) centre (61.136, -79.2443) ccw
  line L130 (47.4058, -83.7785) -> (56.7245, -83.7785)
  arc A117 (45.4858, -80.7902) -> (45.4048, -81.8478) centre (45.9741, -81.3595) ccw
  line L131 (45.4048, -81.8478) -> (46.8366, -83.5169)
  arc A118 (63.7587, -77.9827) -> (64.0117, -77.5275) centre (63.2704, -77.4134) ccw
  arc A119 (46.8366, -83.5169) -> (47.4058, -83.7785) centre (47.4058, -83.0285) ccw
  arc A120 (46.7825, -77.9827) -> (47.0354, -77.5275) centre (46.2942, -77.4134) ccw
  line L132 (47.6202, -78.9593) -> (45.4858, -80.7902)
  line L133 (46.7825, -77.9827) -> (44.648, -79.8136)
  arc A121 (43.5905, -79.7327) -> (44.648, -79.8136) centre (44.1597, -79.2443) ccw
  line L134 (43.5905, -79.7327) -> (42.1587, -78.0636)
  arc A122 (41.9867, -77.4612) -> (42.1587, -78.0636) centre (42.728, -77.5753) ccw
  line L135 (65.0835, -47.7215) -> (50.0835, -47.7215) construction
  line L136 (53.2755, -45.2215) -> (62.5942, -45.2215)
  arc A123 (53.2755, -45.2215) -> (52.7872, -45.4022) centre (53.2755, -45.9715) ccw
  line L137 (52.7872, -45.4022) -> (50.6527, -47.2331)
  arc A124 (50.6527, -47.2331) -> (50.5718, -48.2907) centre (51.141, -47.8024) ccw
  arc A125 (49.4333, -49.2673) -> (48.3757, -49.1864) centre (48.864, -49.7557) ccw
  line L138 (30.3514, -62) -> (29.6486, -67) construction
  line L139 (25.692, -62) -> (35.0107, -62)
  line L140 (24.9893, -67) -> (34.308, -67)
  arc A126 (27.0035, -49.9598) -> (27.5728, -50.2215) centre (27.5728, -49.4715) ccw
  line L141 (37.9646, -51.4725) -> (36.5465, -60.6826)
  arc A127 (38.2175, -51.0173) -> (37.9646, -51.4725) centre (38.7058, -51.5866) ccw
  line L142 (43.0133, -51.5388) -> (41.5952, -60.749)
  line L143 (27.5728, -50.2215) -> (36.8915, -50.2215)
  line L144 (40.352, -49.1864) -> (38.2175, -51.0173)
  arc A128 (41.3422, -61.2041) -> (41.5952, -60.749) centre (40.8539, -60.6349) ccw
  line L145 (41.3422, -61.2041) -> (39.2078, -63.0351)
  arc A129 (38.1502, -62.9541) -> (39.2078, -63.0351) centre (38.7195, -62.4658) ccw
  arc A130 (38.8261, -66.0459) -> (37.7685, -65.9649) centre (38.2568, -66.5342) ccw
  line L146 (38.8261, -66.0459) -> (40.2578, -67.7149)
  line L147 (22.9883, -65.0693) -> (24.42, -66.7383)
  line L148 (21.8498, -66.0459) -> (23.2815, -67.7149)
  arc A131 (23.4535, -68.3174) -> (23.2815, -67.7149) centre (22.7123, -68.2032) ccw
  arc A132 (24.42, -66.7383) -> (24.9893, -67) centre (24.9893, -66.25) ccw
  arc A133 (21.8498, -66.0459) -> (20.7922, -65.9649) centre (21.2805, -66.5342) ccw
  line L149 (20.7922, -65.9649) -> (18.6578, -67.7959)
  arc A134 (18.6578, -67.7959) -> (18.4048, -68.251) centre (19.1461, -68.3651) ccw
  line L150 (18.4048, -68.251) -> (16.9867, -77.4612)
  line L151 (23.4535, -68.3174) -> (22.0354, -77.5275)
  line L152 (25.5718, -48.2907) -> (27.0035, -49.9598)
  arc A135 (26.037, -51.5388) -> (25.865, -50.9364) centre (25.2958, -51.4247) ccw
  line L153 (24.4333, -49.2673) -> (25.865, -50.9364)
  line L154 (23.3757, -49.1864) -> (21.2413, -51.0173)
  line L155 (26.037, -51.5388) -> (24.6189, -60.749)
  arc A136 (21.2413, -51.0173) -> (20.9883, -51.4725) centre (21.7296, -51.5866) ccw
  arc A137 (25.692, -62) -> (25.2037, -62.1807) centre (25.692, -62.75) ccw
  arc A138 (24.3659, -61.2041) -> (24.6189, -60.749) centre (23.8776, -60.6349) ccw
  line L156 (23.945, -48.6981) -> (21.6622, -63.5234) construction
  line L157 (20.9883, -51.4725) -> (19.5702, -60.6826)
  arc A139 (23.0693, -64.0117) -> (22.9883, -65.0693) centre (23.5576, -64.5809) ccw
  line L158 (24.3659, -61.2041) -> (22.2315, -63.0351)
  line L159 (25.2037, -62.1807) -> (23.0693, -64.0117)
  arc A140 (21.1739, -62.9541) -> (22.2315, -63.0351) centre (21.7432, -62.4658) ccw
  arc A141 (35.58, -62.2617) -> (35.0107, -62) centre (35.0107, -62.75) ccw
  arc A142 (36.5465, -60.6826) -> (36.7185, -61.2851) centre (37.2877, -60.7968) ccw
  line L160 (38.1502, -62.9541) -> (36.7185, -61.2851)
  line L161 (35.58, -62.2617) -> (37.0117, -63.9307)
  line L162 (34.7963, -66.8193) -> (36.9307, -64.9883)
  arc A143 (36.9307, -64.9883) -> (37.0117, -63.9307) centre (36.4424, -64.4191) ccw
  arc A144 (19.5702, -60.6826) -> (19.7422, -61.2851) centre (20.3114, -60.7968) ccw
  line L163 (21.1739, -62.9541) -> (19.7422, -61.2851)
  arc A145 (33.963, -77.4612) -> (34.135, -78.0636) centre (34.7042, -77.5753) ccw
  arc A146 (34.308, -67) -> (34.7963, -66.8193) centre (34.308, -66.25) ccw
  line L164 (35.3811, -68.251) -> (33.963, -77.4612)
  arc A147 (35.6341, -67.7959) -> (35.3811, -68.251) centre (36.1224, -68.3651) ccw
  line L165 (35.5667, -79.7327) -> (34.135, -78.0636)
  line L166 (38.7587, -77.9827) -> (36.6243, -79.8136)
  line L167 (40.4298, -68.3174) -> (39.0117, -77.5275)
  line L168 (37.7685, -65.9649) -> (35.6341, -67.7959)
  arc A148 (40.4298, -68.3174) -> (40.2578, -67.7149) centre (39.6886, -68.2032) ccw
  arc A149 (43.0133, -51.5388) -> (42.8413, -50.9364) centre (42.272, -51.4247) ccw
  arc A150 (38.1634, -45.4831) -> (37.5942, -45.2215) centre (37.5942, -45.9715) ccw
  line L169 (38.1634, -45.4831) -> (39.5952, -47.1522)
  arc A151 (39.5142, -48.2098) -> (39.5952, -47.1522) centre (39.0259, -47.6405) ccw
  line L170 (37.3798, -50.0407) -> (39.5142, -48.2098)
  arc A152 (41.4095, -49.2673) -> (40.352, -49.1864) centre (40.8403, -49.7557) ccw
  line L171 (41.4095, -49.2673) -> (42.8413, -50.9364)
  arc A153 (36.8915, -50.2215) -> (37.3798, -50.0407) centre (36.8915, -49.4715) ccw
  arc A154 (23.1085, -78.7785) -> (22.6202, -78.9593) centre (23.1085, -79.5285) ccw
  line L172 (23.1085, -78.7785) -> (32.4272, -78.7785)
  arc A155 (31.7245, -83.7785) -> (32.2128, -83.5978) centre (31.7245, -83.0285) ccw
  arc A156 (32.9965, -79.0402) -> (32.4272, -78.7785) centre (32.4272, -79.5285) ccw
  line L173 (32.2128, -83.5978) -> (34.3473, -81.7669)
  line L174 (32.9965, -79.0402) -> (34.4282, -80.7093)
  arc A157 (34.3473, -81.7669) -> (34.4282, -80.7093) centre (33.859, -81.1976) ccw
  arc A158 (35.5667, -79.7327) -> (36.6243, -79.8136) centre (36.136, -79.2443) ccw
  line L175 (22.4058, -83.7785) -> (31.7245, -83.7785)
  arc A159 (20.4858, -80.7902) -> (20.4048, -81.8478) centre (20.9741, -81.3595) ccw
  line L176 (20.4048, -81.8478) -> (21.8366, -83.5169)
  arc A160 (38.7587, -77.9827) -> (39.0117, -77.5275) centre (38.2704, -77.4134) ccw
  arc A161 (21.8366, -83.5169) -> (22.4058, -83.7785) centre (22.4058, -83.0285) ccw
  arc A162 (21.7825, -77.9827) -> (22.0354, -77.5275) centre (21.2942, -77.4134) ccw
  line L177 (22.6202, -78.9593) -> (20.4858, -80.7902)
  line L178 (21.7825, -77.9827) -> (19.648, -79.8136)
  arc A163 (18.5905, -79.7327) -> (19.648, -79.8136) centre (19.1597, -79.2443) ccw
  line L179 (18.5905, -79.7327) -> (17.1587, -78.0636)
  arc A164 (16.9867, -77.4612) -> (17.1587, -78.0636) centre (17.728, -77.5753) ccw
  line L180 (40.0835, -47.7215) -> (25.0835, -47.7215) construction
  line L181 (28.2755, -45.2215) -> (37.5942, -45.2215)
  arc A165 (28.2755, -45.2215) -> (27.7872, -45.4022) centre (28.2755, -45.9715) ccw
  line L182 (27.7872, -45.4022) -> (25.6527, -47.2331)
  arc A166 (25.6527, -47.2331) -> (25.5718, -48.2907) centre (26.141, -47.8024) ccw
  arc A167 (24.4333, -49.2673) -> (23.3757, -49.1864) centre (23.864, -49.7557) ccw
  point P0 (0, 0)
  point P1 (30, -64.5)
  point P2 (34.5856, -67)
  point P3 (24.6445, -67)
  point P4 (24.5766, -61.0234)
  point P5 (25.4144, -62)
  point P6 (22.5, -64.5)
  point P7 (35.3555, -62)
  point P8 (21.3615, -65.4766)
  point P9 (36.494, -61.0234)
  point P10 (41.5529, -61.0234)
  point P11 (40.4823, -67.9766)
  point P12 (38.3378, -65.4766)
  point P13 (38.6385, -63.5234)
  point P14 (43.0658, -51.1981)
  point P15 (38.0068, -51.1981)
  point P16 (26.0895, -51.1981)
  point P17 (19.5177, -61.0234)
  point P18 (21.0306, -51.1981)
  point P19 (21.9932, -77.8019)
  point P20 (16.9342, -77.8019)
  point P21 (19.0788, -80.3019)
  point P22 (18.4471, -67.9766)
  point P23 (23.506, -67.9766)
  point P24 (22.8309, -78.7785)
  point P25 (32.0021, -83.7785)
  point P26 (32.772, -78.7785)
  point P27 (22.0611, -83.7785)
  point P28 (19.9165, -81.2785)
  point P29 (40.9212, -48.6981)
  point P30 (37.9389, -45.2215)
  point P31 (37.1691, -50.2215)
  point P32 (27.9979, -45.2215)
  point P33 (27.228, -50.2215)
  point P34 (37.5, -64.5)
  point P35 (35.4234, -67.9766)
  point P36 (34.9165, -81.2785)
  point P37 (33.9105, -77.8019)
  point P38 (38.9694, -77.8019)
  point P39 (36.055, -80.3019)
  point P40 (30, -64.5)
  point P41 (0.4144, -62)
  point P42 (5, -64.5)
  point P43 (10.3555, -62)
  point P44 (9.5856, -67)
  point P45 (-0.3555, -67)
  point P46 (11.494, -61.0234)
  point P47 (2.228, -50.2215)
  point P48 (13.0068, -51.1981)
  point P49 (18.0658, -51.1981)
  point P50 (16.5529, -61.0234)
  point P51 (12.1691, -50.2215)
  point P52 (15.9212, -48.6981)
  point P53 (5, -64.5)
  point P54 (13.6385, -63.5234)
  point P55 (12.5, -64.5)
  point P56 (13.3378, -65.4766)
  point P57 (15.4823, -67.9766)
  point P58 (-2.5, -64.5)
  point P59 (-3.6385, -65.4766)
  point P60 (-1.494, -67.9766)
  point P61 (-6.5529, -67.9766)
  point P62 (-8.0658, -77.8019)
  point P63 (-3.0068, -77.8019)
  point P64 (1.0895, -51.1981)
  point P65 (-3.9694, -51.1981)
  point P66 (-0.4234, -61.0234)
  point P67 (-5.4823, -61.0234)
  point P68 (8.9105, -77.8019)
  point P69 (10.4234, -67.9766)
  point P70 (11.055, -80.3019)
  point P71 (13.9694, -77.8019)
  point P72 (12.9389, -45.2215)
  point P73 (7.772, -78.7785)
  point P74 (-2.1691, -78.7785)
  point P75 (7.0021, -83.7785)
  point P76 (9.9165, -81.2785)
  point P77 (-2.9389, -83.7785)
  point P78 (-5.0835, -81.2785)
  point P79 (-5.9212, -80.3019)
  point P80 (2.9979, -45.2215)
  point P81 (50.4144, -62)
  point P82 (55, -64.5)
  point P83 (60.3555, -62)
  point P84 (59.5856, -67)
  point P85 (49.6445, -67)
  point P86 (61.494, -61.0234)
  point P87 (52.228, -50.2215)
  point P88 (63.0068, -51.1981)
  point P89 (68.0658, -51.1981)
  point P90 (66.5529, -61.0234)
  point P91 (62.1691, -50.2215)
  point P92 (65.9212, -48.6981)
  point P93 (55, -64.5)
  point P94 (63.6385, -63.5234)
  point P95 (62.5, -64.5)
  point P96 (63.3378, -65.4766)
  point P97 (65.4823, -67.9766)
  point P98 (47.5, -64.5)
  point P99 (46.3615, -65.4766)
  point P100 (48.506, -67.9766)
  point P101 (43.4471, -67.9766)
  point P102 (41.9342, -77.8019)
  point P103 (46.9932, -77.8019)
  point P104 (51.0895, -51.1981)
  point P105 (46.0306, -51.1981)
  point P106 (49.5766, -61.0234)
  point P107 (44.5177, -61.0234)
  point P108 (58.9105, -77.8019)
  point P109 (60.4234, -67.9766)
  point P110 (61.055, -80.3019)
  point P111 (63.9694, -77.8019)
  point P112 (62.9389, -45.2215)
  point P113 (57.772, -78.7785)
  point P114 (47.8309, -78.7785)
  point P115 (57.0021, -83.7785)
  point P116 (59.9165, -81.2785)
  point P117 (47.0611, -83.7785)
  point P118 (44.9165, -81.2785)
  point P119 (44.0788, -80.3019)
  point P120 (52.9979, -45.2215)
  point P121 (25.4144, -62)
  point P122 (30, -64.5)
  point P123 (35.3555, -62)
  point P124 (34.5856, -67)
  point P125 (24.6445, -67)
  point P126 (36.494, -61.0234)
  point P127 (27.228, -50.2215)
  point P128 (38.0068, -51.1981)
  point P129 (43.0658, -51.1981)
  point P130 (41.5529, -61.0234)
  point P131 (37.1691, -50.2215)
  point P132 (40.9212, -48.6981)
  point P133 (30, -64.5)
  point P134 (38.6385, -63.5234)
  point P135 (37.5, -64.5)
  point P136 (38.3378, -65.4766)
  point P137 (40.4823, -67.9766)
  point P138 (22.5, -64.5)
  point P139 (21.3615, -65.4766)
  point P140 (23.506, -67.9766)
  point P141 (18.4471, -67.9766)
  point P142 (16.9342, -77.8019)
  point P143 (21.9932, -77.8019)
  point P144 (26.0895, -51.1981)
  point P145 (21.0306, -51.1981)
  point P146 (24.5766, -61.0234)
  point P147 (19.5177, -61.0234)
  point P148 (33.9105, -77.8019)
  point P149 (35.4234, -67.9766)
  point P150 (36.055, -80.3019)
  point P151 (38.9694, -77.8019)
  point P152 (37.9389, -45.2215)
  point P153 (32.772, -78.7785)
  point P154 (22.8309, -78.7785)
  point P155 (32.0021, -83.7785)
  point P156 (34.9165, -81.2785)
  point P157 (22.0611, -83.7785)
  point P158 (19.9165, -81.2785)
  point P159 (19.0788, -80.3019)
  point P160 (27.9979, -45.2215)
  dimension "d109" = 1.5
  dimension "d110" = 5
  dimension "d111" = 5
  dimension "d112" = 15
  dimension "d113" = 15
  dimension "d114" = 0.75
  dimension "d115" = 16.9763
  dimension "d116" = 16.9763
  dimension "d117" = 16.9763
  dimension "d119" = 8
  dimension "d122" = 25
  dimension "d125" = 25
  constraints: 362 end point, 336 point on circle, 336 point on line, 168 centre point, 24 tangent, 11 equal radius, 7 collinear, 6 midpoint, 5 parallel, 4 coincident, 4 horizontal, 1 perpendicular, 959 other
  measures "d109" distance between parallel lines of L30 L35
  measures "d110" distance between parallel lines of L33 L31
  measures "d111" distance between parallel lines of L11 L13
  measures "d112" distance of L32.start L32.end
  measures "d113" distance of L12.start L12.end
  measures "d114" radius of A28
  measures "d115" distance of L30.start L25.start
  measures "d116" distance of L30.start L20.start
  measures "d117" distance of L31.start L5.start
  measures "d119" angle of L46 L0
  measures "d122" distance of point (25.414, -62) point (0.414, -62)
  measures "d125" distance of point (25.414, -62) point (50.414, -62)
extrude "Extrusion5" cut sketch "Sketch14" against normal blind 0.5 contours L4 A3 L14 A12 L13 A26 L29 A28 L30 A27 L11 A1 | L7 A5 L9 A8 L10 A9 L27 A23 L25 A6 L8 A4 | L6 A36 L42 A41 L43 A40 L44 A39 L41 A35 L38 A10 | L17 A15 L19 A16 L20 A17 L18 A18 L15 A14 L16 A13 | L22 A21 L23 A22 L24 A20 L21 A37 L40 A38 L39 A19 | L26 A25 L28 A24 L33 A31 L35 A32 L34 A30 L31 A29 | L49 A57 L71 A59 L72 A62 L50 A48 L57 A55 L69 A53 | L62 A82 L92 A81 L91 A66 L79 A67 L80 A69 L53 A42 | A43 L54 A68 L81 A65 L52 A44 L55 A45 L70 A58 L51 | L58 A47 L61 A78 L88 A79 L89 A80 L60 A50 L59 A49 | L82 A72 L84 A73 L83 A71 L85 A77 L86 A75 L87 A70 | L94 A99 L116 A101 L117 A104 L95 A90 L102 A97 L114 A95 | L107 A124 L137 A123 L136 A108 L124 A109 L125 A111 L98 A84 | A85 L99 A110 L126 A107 L97 A86 L100 A87 L115 A100 L96 | L103 A89 L106 A120 L133 A121 L134 A122 L105 A92 L104 A91 | L127 A114 L129 A115 L128 A113 L130 A119 L131 A117 L132 A112
pattern_circular "Circular Pattern1" count 2 over 360 about axis through (30, 0, 102) along (0, 0, -1) of "Extrusion5"
equation "\"d78\" = d70"
equation "\"d79\" = d70"
body "Solid1"
